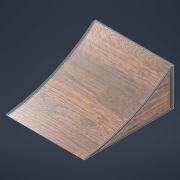
# Autodesk Inventor part: McCrea_rampa_walle
Saved by Autodesk Inventor 2022 (Build 260153000, 153)
## iProperties
Created: 2022-02-12
Part Number: McCrea_rampa_walle
Material: Generic
Document SubType Name: Modeling
Designer: MatusBarany
Density: 1 g/cm^3
Appearance: Smooth - Black
Author: MatusBarany
Autodesk Inventor part; units mm, degrees
ref_plane "YZ Plane" through (0, 0, 0) normal (1, 0, 0) x (0, 1, 0)
ref_plane "XZ Plane" through (0, 0, 0) normal (0, 1, 0) x (-1, 0, 0)
ref_plane "XY Plane" through (0, 0, 0) normal (0, 0, 1) x (1, 0, 0)
sketch "Sketch1" plane through (0, 0, 0) normal (1, 0, 0) x (0, 1, 0)
  line L0 (-23.4551, 209.3237) -> (-23.4551, -140.6763)
  line L1 (-23.4551, -140.6763) -> (126.5449, -140.6763)
  arc A0 (-23.4551, 209.3237) -> (126.5449, -140.6763) centre (632.3907, 283.2577) ccw
  point P0 (0, 0)
  dimension "d0" = 350
  dimension "d1" = 150
  dimension "d2" = 660
  constraints: 4 end point, 2 point on circle, 1 centre point, 1 horizontal, 1 vertical
  measures "d0" distance of L0.start L0.end
  measures "d1" distance of L0.end L1.end
  measures "d2" radius of A0
extrude "Extrusion1" add sketch "Sketch1" along normal blind 300
ref_plane "Work Plane1" through (150, 0, 0) normal (1, 0, 0) x (0, 0, -1)
sketch "Sketch2" plane through (300, 0, 0) normal (1, 0, 0) x (0, 0, -1)
  line L0 (140.6763, -23.4551) -> (140.6763, 126.5449) projected
  arc A0 (-209.3237, -23.4551) -> (140.6763, 126.5449) centre (-283.2577, 632.3907) ccw projected
  line L1 (-209.3237, -23.4551) -> (140.6763, -23.4551) projected
  line L2 (135.6763, 115.9419) -> (135.6763, -18.4551)
  line L3 (135.6763, -18.4551) -> (-146.7854, -18.4551)
  arc A1 (-146.7854, -18.4551) -> (135.6763, 115.9419) centre (-283.2577, 632.3907) ccw
  point P0 (0, 0)
  dimension "d6" = 5
  constraints: 4 end point, 2 point on circle, 1 centre point, 2 other
  measures "d6" distance between parallel lines of L0 L2
extrude "Extrusion2" add sketch "Sketch2" along normal blind 5
sketch "Sketch3" plane through (0, -23.4551, -140.6763) normal (0, 0, -1) x (-1, 0, 0)
  line L0 (0, 0) -> (0, 150) projected
  line L1 (0, 150) -> (-305, 150) projected
  line L2 (-305, 0) -> (-305, 150) projected
  line L3 (0, 0) -> (-305, 0) projected
  line L4 (-300, 145) -> (-5, 145)
  line L5 (-5, 145) -> (-5, 5)
  line L6 (-5, 5) -> (-300, 5)
  line L7 (-300, 5) -> (-300, 145)
  line L8 (-305, 0) -> (-305, 150) projected
  line L9 (-305, 150) -> (-305, 0) projected
  line L10 (-305, 139.397) -> (-305, 5) projected
  line L11 (-305, 5) -> (-305, 139.397) projected
  point P0 (0, 23.4551)
  dimension "d9" = 5
  constraints: 8 end point, 3 other
  measures "d9" distance between parallel lines of L1 L4
extrude "Extrusion3" cut sketch "Sketch3" against normal blind 5 contours L4 L5 L6 L7
sketch "Sketch4" plane through (305, 0, 0) normal (1, 0, 0) x (0, 0, -1)
  arc A0 (-209.3237, -23.4551) -> (140.6763, 126.5449) centre (-283.2577, 632.3907) ccw projected
  arc A1 (-209.6598, -20.474) -> (138.7493, 128.8442) centre (-283.2577, 632.3907) ccw
  line L0 (140.6763, 126.5449) -> (138.7493, 128.8442)
  line L1 (-209.3237, -23.4551) -> (-209.6598, -20.474)
  point P0 (0, 0)
  point P1 (140.6763, 126.5449)
  dimension "d12" = 3
  constraints: 4 end point, 2 point on circle, 1 centre point
  measures "d12" radial gap between concentric circles of A1 A0
extrude "Extrusion4" add sketch "Sketch4" against normal blind 5
sketch "Sketch5" plane through (305, -23.4551, -140.6763) normal (0, 0, -1) x (-1, 0, 0)
  line L0 (300, 145) -> (300, 5) projected
  line L1 (300, 5) -> (5, 5) projected
  line L2 (5, 5) -> (5, 145) projected
  line L3 (5, 145) -> (300, 145) projected
  line L4 (305, 150) -> (5, 150) projected
  line L5 (5, 150) -> (0, 150) projected
  line L6 (0, 0) -> (0, 150) projected
  line L7 (305, 0) -> (305, 150) projected
  line L8 (305, 0) -> (0, 0) projected
  point P0 (305, 23.4551)
extrude "Extrusion5" add sketch "Sketch5" along normal blind 5
chamfer "Chamfer1" distance 3.6 angle 40 1 edges at (302.5, 128.8442, -138.7493) measured on face at (302.5, 128.5231, -138.366)
mirror "Mirror3" about plane through (150, 0, 0) normal (1, 0, 0) of "Extrusion2", "Extrusion4", "Extrusion5", "Chamfer1"
body "Solid1"
